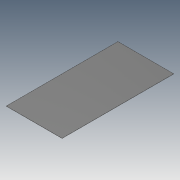
# Autodesk Inventor part: Panel_A
Saved by Autodesk Inventor 2020 (Build 240168000, 168)
## iProperties
Created: 2021-02-24
Part Number: Panel_A
Material: アルミニウム 6061
Document SubType Name: Modeling
Designer: magnarecta
Density: 2.7 g/cm^3
Appearance: 細かい テクスチャ - 黒
Author: magnarecta
Autodesk Inventor part; units mm, degrees
ref_plane "YZ Plane" through (0, 0, 0) normal (1, 0, 0) x (0, 1, 0)
ref_plane "XZ Plane" through (0, 0, 0) normal (0, 1, 0) x (-1, 0, 0)
ref_plane "XY Plane" through (0, 0, 0) normal (0, 0, 1) x (1, 0, 0)
sketch "スケッチ1" plane through (0, 0, 0) normal (0, 1, 0) x (-1, 0, 0)
  line L0 (-375, -750) -> (375, -750)
  line L1 (375, -750) -> (375, 750)
  line L2 (375, 750) -> (-375, 750)
  line L3 (-375, 750) -> (-375, -750)
  line L4 (-375, -750) -> (375, 750) construction
  line L5 (375, -750) -> (-375, 750) construction
  point P0 (0, 0)
  dimension "d0" = 1500
  dimension "d1" = 750
  constraints: 12 end point, 2 midpoint, 2 parallel, 1 horizontal, 1 perpendicular
  measures "d0" distance of L0.end L1.end
  measures "d1" distance of L1.end L2.end
extrude "押し出し1" add sketch "スケッチ1" along normal blind 2
